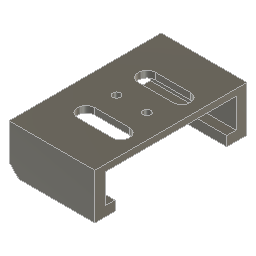
Крепление аккамулятора Bosch_ver2 (Autodesk Fusion 360 design; units mm, degrees)
Autodesk Fusion 360 part; units mm, degrees
sketch "Sketch1" plane through (0, 0, 0) normal (0, 0, 1) x (1, 0, 0)
  line L0 (30, 25.7) -> (-30, 25.7)
  line L1 (-30, 25.7) -> (-30, -25.7)
  line L2 (-30, -25.7) -> (30, -25.7)
  line L3 (30, -25.7) -> (30, 25.7)
  line L4 (30, -30) -> (-30, -30)
  line L5 (-30, -35) -> (-30, 35)
  line L6 (-30, 30) -> (30, 30)
  line L7 (30, 30) -> (30, -30)
  line L8 (-30, 35) -> (27, 35)
  line L9 (35, 27) -> (35, -27)
  line L10 (-30, -35) -> (27, -35)
  arc A0 (35, 27) -> (27, 35) centre (27, 27) ccw
  arc A1 (27, -35) -> (35, -27) centre (27, -27) ccw
  circle A2 centre (-20, 0) radius 1.75
  line L11 (-19.9675, 10) -> (-4, 10)
  arc A3 (-4, 10) -> (-4, 18) centre (-4, 14) ccw
  line L12 (-4, 18) -> (-19.9675, 18)
  arc A4 (-19.9675, 18) -> (-19.9675, 10) centre (-19.9675, 14) ccw
  line L13 (-19.9675, 14) -> (-4, 14) construction
  line L14 (1.75, 0) -> (22.5, 0)
  line L15 (-19.9675, -10) -> (-4, -10)
  arc A5 (-19.9675, -10) -> (-19.9675, -18) centre (-19.9675, -14) ccw
  line L16 (-4, -18) -> (-19.9675, -18)
  arc A6 (-4, -18) -> (-4, -10) centre (-4, -14) ccw
  circle A7 centre (-6, 0) radius 1.75
  dimension "d1" = 60
  dimension "d2" = 51.4
  dimension "d3" = 60
  dimension "d6" = 8
  dimension "d15" = 3.5
  dimension "d37" = 3.5
  constraint horizontal L0
  constraint perpendicular L0 L1
  constraint parallel L0 L2
  constraint parallel L1 L3
  constraint horizontal L4
  constraint perpendicular L4 L5
  constraint parallel L4 L6
  constraint parallel L5 L7
  constraint coincident L6.start L5
  constraint coincident L4.end L5
  constraint tangent L9 A0
  constraint tangent L8 A0
  constraint tangent L10 A1
  constraint tangent L9 A1
  constraint equal A0 A1
  constraint tangent L11 A3
  constraint tangent A3 L12
  constraint parallel L11 L12
  constraint tangent L12 A4
  constraint tangent L11 A4
  constraint horizontal L13
  constraint symmetric L11.start L14 L15.start
  constraint symmetric L11.end L14 L15.end
  constraint symmetric A3.end L14 L16.start
  constraint symmetric L12.end L14 A5.end
  constraint symmetric A3 L14 A6
  constraint symmetric A4 L14 A5
  measures "d1" distance of L1.end L2.end
  measures "d2" distance of L0.end L1.end
  measures "d3" distance of L4.end L6.start
  measures "d6" radius of A0
  measures "d15" diameter of A2
  measures "d37" diameter of A7
extrude "Extrude1" add sketch "Sketch1" along normal blind 4.5 contours L3 L4 L5 L6 L7 L8 L9 L10 A0 A1 | L0 L5 L6 L7 | L2 L4 L5 L7
extrude "Extrude2" add sketch "Sketch1" along normal blind 18 contours L3 L4 L5 L6 L7 L8 L9 L10 A0 A1
extrude "Extrude3" add sketch "Sketch1" along normal blind 21 and the other way blind -18
sketch "Sketch2" plane through (0, -35, 0) normal (0, -1, 0) x (1, 0, 0)
  line L0 (-30, 0) -> (27, 0)
  line L1 (27, 0) -> (27, 21)
  line L2 (27, 21) -> (-30, 21)
  line L3 (-30, 21) -> (-30, 0)
  line L4 (-30, 0) -> (-34.45, 0)
  line L5 (-34.45, 0) -> (-34.45, 4.55)
  line L6 (-30, 0) -> (-30.316, 0.3196)
  line L7 (-30.316, 0.3196) -> (-34.45, 4.55)
  line L8 (-34.45, 4.55) -> (-34.45, 21)
  line L9 (-34.45, 21) -> (-30, 21)
  line L10 (-30, 0) -> (-30, 5.5)
  line L11 (-30, 5.5) -> (-34.45, 5.5)
  line L12 (-34.45, 4.55) -> (-29.5, 4.55)
  dimension "d17" = 4.45
  dimension "d18" = 4.55
  dimension "d25" = 5.5
  constraint coincident L0.start L3.end
  constraint perpendicular L3 L4
  constraint perpendicular L4 L5
  constraint parallel L5 L8
  constraint coincident L2.end L3.start
  constraint perpendicular L3 L9
  constraint perpendicular L4 L10
  constraint coincident L8 L11.end
  constraint perpendicular L8 L11
  constraint perpendicular L3 L12
  measures "d17" distance of L0.start L4.end
  measures "d18" distance of L4.end L5.end
  measures "d25" distance of L0.start L10.end
extrude "Extrude4" add sketch "Sketch2" against normal blind 5 contours L3 L6 L7 L10 L12 | L3 L8 L10 L11 L12 | L3 L8 L9 L11
extrude "Extrude5" add sketch "Sketch2" along normal blind -70 and the other way blind 65 contours L3 L6 L7 L10 L12 | L3 L8 L10 L11 L12 | L3 L8 L9 L11
extrude "Extrude6" add sketch "Sketch2" against normal blind 9.3 contours L3 L6 L7 L10 L12
extrude "Extrude7" add sketch "Sketch2" along normal blind -65 and the other way blind 60.7 contours L3 L6 L7 L10 L12
extrude "Extrude8" add 1 faces at (-30, -10, 19) along direction (-1, 0, 0) blind 4.45
extrude "Extrude9" cut 2 faces at (-32.9667, -28.5667, 4.55) (-32.9667, 27.1333, 4.55) along direction (0, 0, -1) blind 0.05
sketch "Sketch3" plane through (0, 0, 21) normal (0, 0, 1) x (-1, 0, 0)
  circle A0 centre (20, 0) radius 1.75
  arc A1 (19.9675, -18) -> (19.9675, -10) centre (19.9675, -14) ccw
  line L0 (19.9675, -18) -> (4, -18)
  arc A2 (4, -10) -> (4, -18) centre (4, -14) ccw
  line L1 (4, -10) -> (19.9675, -10)
  arc A3 (19.9675, 10) -> (19.9675, 18) centre (19.9675, 14) ccw
  line L2 (19.9675, 10) -> (4, 10)
  arc A4 (4, 18) -> (4, 10) centre (4, 14) ccw
  line L3 (4, 18) -> (19.9675, 18)
  line L4 (34.45, 35) -> (-27, 35)
  arc A5 (-27, 35) -> (-35, 27) centre (-27, 27) ccw
  line L5 (-35, 27) -> (-35, -27)
  arc A6 (-35, -27) -> (-27, -35) centre (-27, -27) ccw
  line L6 (-27, -35) -> (34.45, -35)
  line L7 (34.45, -35) -> (34.45, 35)
  line L8 (-5, -40) -> (-40, -40)
  line L9 (-40, -40) -> (-40, 40)
  line L10 (-40, 40) -> (-5, 40)
  line L11 (-5, 40) -> (-5, -40)
  circle A7 centre (6, 0) radius 1.75
  constraint horizontal L8
  constraint vertical L9
  constraint horizontal L10
  constraint vertical L11
extrude "Extrude10" cut sketch "Sketch3" against normal blind 40 contours L4 A5 L5 A6 L6 L11 | L4 A5 L5 A6 L6 L8 L9 L10 L11
